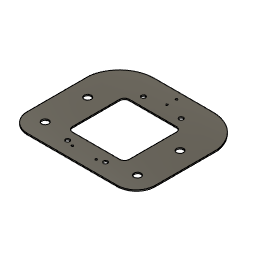
Knob plate (Autodesk Fusion 360 design; units mm, degrees)
Autodesk Fusion 360 part; units mm, degrees
note: some values were not read from the file. Set by a fixed rule: which sketch regions a step uses.
sketch "Esquisse1" plane through (0, 0, 0) normal (0, 0, 1) x (1, 0, 0)
  line L0 (-135, 125) -> (135, 125)
  line L1 (135, 125) -> (135, -125)
  line L2 (135, -125) -> (-135, -125)
  line L3 (-135, -125) -> (-135, 125)
  line L4 (0, 1.75) -> (0, 22.5)
  line L5 (1.75, 0) -> (22.5, 0)
  dimension "d1" = 270
  dimension "d2" = 250
  constraint horizontal L0
  constraint vertical L1
  constraint horizontal L2
  constraint vertical L3
  constraint symmetric L1 L3 L4
  constraint symmetric L0 L2 L5
  measures "d1" distance of L0.start L0.end
  measures "d2" distance of L0.end L1.end
extrude "Face1" add sketch "Esquisse1" along normal blind 2.5
sketch "Esquisse2" plane through (0, 0, 2.5) normal (0, 0, 1) x (-1, 0, 0)
  line L0 (60, -60) -> (-60, -60)
  line L1 (-60, -60) -> (-60, 60)
  line L2 (-60, 60) -> (60, 60)
  line L3 (60, 60) -> (60, -60)
  line L4 (0, -1.75) -> (0, -22.5)
  line L5 (-1.75, 0) -> (-22.5, 0)
  dimension "d5" = 120
  dimension "d6" = 120
  constraint horizontal L0
  constraint vertical L1
  constraint horizontal L2
  constraint vertical L3
  constraint symmetric L1 L3 L4
  constraint symmetric L0 L2 L5
  measures "d5" distance of L0.start L0.end
  measures "d6" distance of L0.end L1.end
extrude "Extrusion7" cut sketch "Esquisse2" against normal through all
fillet "Congé3" radius 10 4 edges at (-60, 60, 1.25) (60, 60, 1.25) (60, -60, 1.25) (-60, -60, 1.25)
sketch "Esquisse3" plane through (0, 0, 2.5) normal (0, 0, 1) x (-1, 0, 0)
  circle A0 centre (97.5, -20) radius 7.5
  circle A1 centre (-97.5, -20) radius 7.5
  circle A2 centre (97.5, 70) radius 7.5
  circle A3 centre (-97.5, 70) radius 7.5
  line L0 (135, 125) -> (-135, 125)
  line L1 (60, 50) -> (60, -50)
  line L2 (0, -1.75) -> (0, -22.5)
  line L3 (-50, 60) -> (50, 60)
  line L4 (-1.75, 0) -> (-22.5, 0)
  line L5 (50, -60) -> (-50, -60)
  dimension "d14" = 15
  dimension "d16" = 15
  dimension "d52" = 37.5
  dimension "d53" = 37.5
  dimension "d80" = 10
  dimension "d95" = 90
  constraint symmetric A2 A3 L2
  constraint symmetric A0 A1 L2
  measures "d14" diameter of A0
  measures "d16" diameter of A2
  measures "d52" distance of A2.centre L1
  measures "d53" distance of A0.centre L1
  measures "d80" distance of A2.centre L3
  measures "d95" distance of A0.centre A2.centre
extrude "Extrusion8" cut sketch "Esquisse3" against normal through all
sketch "Esquisse4" plane through (0, 0, 2.5) normal (0, 0, 1) x (-1, 0, 0)
  circle A0 centre (40, -80) radius 4.5
  circle A1 centre (-40, -80) radius 4.5
  circle A2 centre (40, 80) radius 4.5
  circle A3 centre (-40, 80) radius 4.5
  line L0 (-1.75, 0) -> (-22.5, 0)
  line L1 (50, -60) -> (-50, -60)
  line L2 (135, -125) -> (135, 125)
  line L3 (0, -1.75) -> (0, -22.5)
  dimension "d23" = 9
  dimension "d55" = 20
  dimension "d83" = 40
  constraint symmetric A0 A2 L0
  constraint symmetric A1 A3 L0
  constraint symmetric A0 A1 L3
  measures "d23" diameter of A0
  measures "d55" distance of A0.centre L1
  measures "d83" distance of A0.centre L3
extrude "Extrusion9" cut sketch "Esquisse4" against normal through all
sketch "Esquisse8" plane through (0, 0, 2.5) normal (0, 0, 1) x (-1, 0, 0)
  line L0 (135, -125) -> (135, 125)
  line L1 (135, 125) -> (-135, 125)
  line L2 (-135, 125) -> (-135, -125)
  line L3 (-135, -125) -> (135, -125)
  line L4 (60, 50) -> (60, -50)
  arc A0 (50, -60) -> (60, -50) centre (50, -50) ccw
  line L5 (50, -60) -> (-50, -60)
  arc A1 (-60, -50) -> (-50, -60) centre (-50, -50) ccw
  line L6 (-60, -50) -> (-60, 50)
  arc A2 (-50, 60) -> (-60, 50) centre (-50, 50) ccw
  line L7 (-50, 60) -> (50, 60)
  arc A3 (60, 50) -> (50, 60) centre (50, 50) ccw
  circle A4 centre (-97.5, 70) radius 7.5
  circle A5 centre (97.5, -20) radius 7.5
  circle A6 centre (-97.5, -20) radius 7.5
  circle A7 centre (97.5, 70) radius 7.5
  circle A8 centre (-40, -80) radius 4.5
  circle A9 centre (-40, 80) radius 4.5
  circle A10 centre (40, -80) radius 4.5
  circle A11 centre (40, 80) radius 4.5
  line L8 (135, 110) -> (-135, 110)
  line L9 (-135, 110) -> (-135, 125)
  line L10 (-135, 125) -> (135, 125)
  line L11 (135, 125) -> (135, 110)
  dimension "d68" = 50
  constraint horizontal L8
  constraint vertical L9
  constraint horizontal L10
  constraint vertical L11
  constraint coincident L2 L1.end
  constraint coincident L0 L8.start
  constraint collinear L1 L10
  measures "d68" distance of L7 L8
extrude "Extrusion12" cut sketch "Esquisse8" against normal through all contours L0 L1 L2 L8 L9 L10 L11
sketch "Esquisse10" plane through (0, 0, 2.5) normal (0, 0, 1) x (-1, 0, 0)
  circle A0 centre (40, 80) radius 4.5
  circle A1 centre (40, -80) radius 4.5
  circle A2 centre (-40, 80) radius 4.5
  circle A3 centre (-40, -80) radius 4.5
  circle A4 centre (97.5, 70) radius 7.5
  circle A5 centre (-97.5, -20) radius 7.5
  circle A6 centre (97.5, -20) radius 7.5
  circle A7 centre (-97.5, 70) radius 7.5
  line L0 (60, 50) -> (60, -50)
  arc A8 (50, -60) -> (60, -50) centre (50, -50) ccw
  line L1 (50, -60) -> (-50, -60)
  arc A9 (-60, -50) -> (-50, -60) centre (-50, -50) ccw
  line L2 (-60, -50) -> (-60, 50)
  arc A10 (-50, 60) -> (-60, 50) centre (-50, 50) ccw
  line L3 (-50, 60) -> (50, 60)
  arc A11 (60, 50) -> (50, 60) centre (50, 50) ccw
  line L4 (-135, 110) -> (-135, -125)
  line L5 (-135, -125) -> (135, -125)
  line L6 (135, -125) -> (135, 110)
  line L7 (135, 110) -> (-135, 110)
  arc A12 (62, -125) -> (135, -62) centre (62, -51.2063) ccw
  line L8 (0, -1.75) -> (0, -22.5)
  arc A13 (-135, -62) -> (-62, -125) centre (-62, -51.2063) ccw
  dimension "d77" = 2
  dimension "d78" = 2
  constraint tangent L5 A12
  constraint coincident L5 A12.start
  constraint coincident L6 A12.end
  constraint symmetric A12.end L8 A13.start
  constraint symmetric A12.start L8 A13.end
  constraint symmetric A12 L8 A13
  measures "d77" distance of L0 A12.start
  measures "d78" distance of L1 A12.end
extrude "Extrusion14" cut sketch "Esquisse10" against normal through all contours L4 L5 A13 | L5 L6 A12
sketch "Esquisse11" plane through (0, 0, 2.5) normal (0, 0, 1) x (-1, 0, 0)
  arc A0 (-135, -62) -> (-62, -125) centre (-62, -51.2063) ccw
  line L0 (-62, -125) -> (62, -125)
  arc A1 (62, -125) -> (135, -62) centre (62, -51.2063) ccw
  line L1 (135, -62) -> (135, 110)
  line L2 (135, 110) -> (-135, 110)
  line L3 (-135, 110) -> (-135, -62)
  circle A2 centre (40, 80) radius 4.5
  circle A3 centre (40, -80) radius 4.5
  circle A4 centre (-40, 80) radius 4.5
  circle A5 centre (-40, -80) radius 4.5
  circle A6 centre (97.5, 70) radius 7.5
  circle A7 centre (-97.5, -20) radius 7.5
  circle A8 centre (97.5, -20) radius 7.5
  circle A9 centre (-97.5, 70) radius 7.5
  line L4 (60, 50) -> (60, -50)
  arc A10 (50, -60) -> (60, -50) centre (50, -50) ccw
  line L5 (50, -60) -> (-50, -60)
  arc A11 (-60, -50) -> (-50, -60) centre (-50, -50) ccw
  line L6 (-60, -50) -> (-60, 50)
  arc A12 (-50, 60) -> (-60, 50) centre (-50, 50) ccw
  line L7 (-50, 60) -> (50, 60)
  arc A13 (60, 50) -> (50, 60) centre (50, 50) ccw
  circle A14 centre (0, -110) radius 2
  circle A15 centre (0, -90) radius 2
  line L8 (0, -1.75) -> (0, -22.5)
  circle A16 centre (0, -90) radius 2
  dimension "d84" = 4
  dimension "d85" = 4
  dimension "d87" = 20
  dimension "d88" = 15
  constraint symmetric A15 L8 A16
  constraint coincident A15.centre L8
  measures "d84" diameter of A14
  measures "d85" diameter of A15
  measures "d87" distance of A14.centre A15.centre
  measures "d88" distance of L0 A14.centre
extrude "Extrusion15" cut sketch "Esquisse11" against normal through all contours A14 | A15 A16
sketch "Esquisse12" plane through (0, 0, 2.5) normal (0, 0, 1) x (-1, 0, 0)
  circle A0 centre (0, -110) radius 2
  arc A1 (-135, -62) -> (-62, -125) centre (-62, -51.2063) ccw
  line L0 (-62, -125) -> (62, -125)
  arc A2 (62, -125) -> (135, -62) centre (62, -51.2063) ccw
  line L1 (135, -62) -> (135, 110)
  line L2 (135, 110) -> (-135, 110)
  line L3 (-135, 110) -> (-135, -62)
  circle A3 centre (40, 80) radius 4.5
  circle A4 centre (40, -80) radius 4.5
  circle A5 centre (-40, 80) radius 4.5
  circle A6 centre (-40, -80) radius 4.5
  circle A7 centre (97.5, 70) radius 7.5
  circle A8 centre (-97.5, -20) radius 7.5
  circle A9 centre (97.5, -20) radius 7.5
  circle A10 centre (-97.5, 70) radius 7.5
  line L4 (60, 50) -> (60, -50)
  arc A11 (50, -60) -> (60, -50) centre (50, -50) ccw
  line L5 (50, -60) -> (-50, -60)
  arc A12 (-60, -50) -> (-50, -60) centre (-50, -50) ccw
  line L6 (-60, -50) -> (-60, 50)
  arc A13 (-50, 60) -> (-60, 50) centre (-50, 50) ccw
  line L7 (-50, 60) -> (50, 60)
  arc A14 (60, 50) -> (50, 60) centre (50, 50) ccw
  circle A15 centre (25, 85) radius 2
  line L8 (0, -1.75) -> (0, -22.5)
  circle A16 centre (-25, 85) radius 2
  circle A17 centre (0, -90) radius 2
  dimension "d91" = 4
  dimension "d93" = 50
  constraint symmetric A15 L8 A16
  measures "d91" diameter of A15
  measures "d93" distance of A15.centre A16.centre
extrude "Extrusion16" cut sketch "Esquisse12" against normal through all contours A15 | A16
fillet "Congé5" radius 40 2 edges at (135, -110, 1.25) (-135, -110, 1.25)
